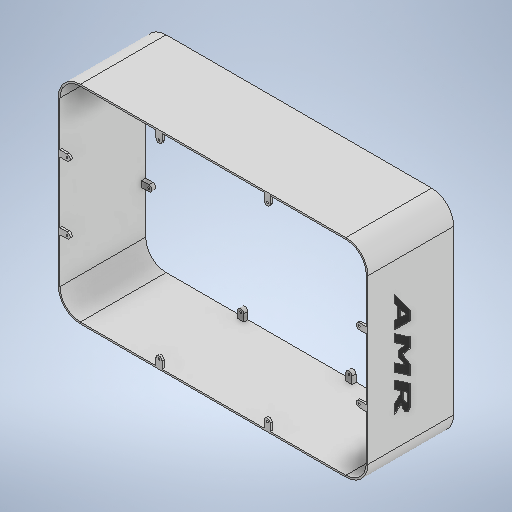
# Autodesk Inventor part: product
Saved by Autodesk Inventor 2025 (Build 290162000, 162)
## iProperties
Created: 2025-10-14
Part Number: product
Material: Generic
Document SubType Name: Modeling
Designer: hp
Density: 1 g/cm^3
Appearance: Default
Author: hp
Autodesk Inventor part; units mm, degrees
ref_plane "YZ Plane" through (0, 0, 0) normal (1, 0, 0) x (0, 1, 0)
ref_plane "XZ Plane" through (0, 0, 0) normal (0, 1, 0) x (-1, 0, 0)
ref_plane "XY Plane" through (0, 0, 0) normal (0, 0, 1) x (1, 0, 0)
sketch "Sketch1" plane through (0, 0, 0) normal (0, 0, 1) x (1, 0, 0)
  line L0 (-325, 250) -> (325, 250)
  line L1 (375, 200) -> (375, -200)
  line L2 (325, -250) -> (-325, -250)
  line L3 (-375, -200) -> (-375, 200)
  line L4 (-375, 250) -> (375, -250) construction
  line L5 (375, 250) -> (-375, -250) construction
  arc A0 (-325, 250) -> (-375, 200) centre (-325, 200) ccw
  arc A1 (-375, -200) -> (-325, -250) centre (-325, -200) ccw
  arc A2 (375, 200) -> (325, 250) centre (325, 200) ccw
  arc A3 (325, -250) -> (375, -200) centre (325, -200) ccw
  line L6 (325, 254) -> (-325, 254)
  arc A4 (-325, 254) -> (-379, 200) centre (-325, 200) ccw
  line L7 (-379, 200) -> (-379, -200)
  arc A5 (-379, -200) -> (-325, -254) centre (-325, -200) ccw
  line L8 (-325, -254) -> (325, -254)
  arc A6 (325, -254) -> (379, -200) centre (325, -200) ccw
  line L9 (379, -200) -> (379, 200)
  arc A7 (379, 200) -> (325, 254) centre (325, 200) ccw
  line L10 (-379, 200) -> (-375, 200)
  line L11 (-375, -200) -> (-379, -200)
  line L12 (379, 200) -> (375, 200)
  line L13 (379, -200) -> (375, -200)
  point P0 (0, 0)
  dimension "d66" = 5
  dimension "d0" = 750
  dimension "d2" = 50
  dimension "d3" = 50
  dimension "d4" = 4
  dimension "d75" = 500
  constraints: 28 end point, 16 point on circle, 9 point on line, 8 centre point, 8 tangent, 6 parallel, 3 perpendicular, 2 equal radius, 2 midpoint, 1 horizontal, 7 other
  measures "d0" distance of L4.end L5.end
  measures "d2" radius of A0
  measures "d3" radius of A3
  measures "d4" distance between parallel lines of L0 L6
  measures "d75" distance between parallel lines of L0 L2
extrude "Extrusion1" add sketch "Sketch1" along normal blind 210 contours A0 L10 A4 L6 A7 L12 A2 L0 | L3 L11 L7 L10 | L12 L9 L13 L1 | A1 L2 A3 L13 A6 L8 A5 L11
sketch "Sketch2" plane through (0, 0, 210) normal (0, 0, 1) x (1, 0, 0)
  line L0 (-325, 250) -> (325, 250) projected
  line L1 (-140, 250) -> (-125, 250)
  line L2 (-125, -250) -> (-140, -250)
  line L3 (125, 250) -> (140, 250)
  line L4 (140, -250) -> (125, -250)
  line L5 (-375, -200) -> (-375, 200) projected
  line L6 (375, 90) -> (375, 75)
  line L7 (-375, 75) -> (-375, 90)
  line L8 (375, 200) -> (375, -200) projected
  line L9 (375, -75) -> (375, -90)
  line L10 (325, -250) -> (-325, -250) projected
  line L11 (125, 232.5) -> (125, 250)
  line L12 (140, 250) -> (140, 232.5)
  line L13 (-125, 250) -> (-125, 232.5)
  line L14 (-140, 232.5) -> (-140, 250)
  line L15 (-375, 90) -> (-357.5, 90)
  line L16 (-357.5, 75) -> (-375, 75)
  line L17 (-375, -75) -> (-357.5, -75)
  line L18 (-357.5, -90) -> (-375, -90)
  line L19 (-140, -250) -> (-140, -232.5)
  line L20 (-125, -232.5) -> (-125, -250)
  line L21 (140, -232.5) -> (140, -250)
  line L22 (125, -250) -> (125, -232.5)
  line L23 (357.5, -75) -> (375, -75)
  line L24 (375, -90) -> (357.5, -90)
  line L25 (357.5, 90) -> (375, 90)
  line L26 (375, 75) -> (357.5, 75)
  arc A0 (-140, 232.5) -> (-125, 232.5) centre (-132.5, 232.5) ccw
  arc A1 (125, 232.5) -> (140, 232.5) centre (132.5, 232.5) ccw
  arc A2 (-357.5, 75) -> (-357.5, 90) centre (-357.5, 82.5) ccw
  arc A3 (-357.5, -90) -> (-357.5, -75) centre (-357.5, -82.5) ccw
  arc A4 (-125, -232.5) -> (-140, -232.5) centre (-132.5, -232.5) ccw
  arc A5 (140, -232.5) -> (125, -232.5) centre (132.5, -232.5) ccw
  arc A6 (357.5, -75) -> (357.5, -90) centre (357.5, -82.5) ccw
  arc A7 (357.5, 90) -> (357.5, 75) centre (357.5, 82.5) ccw
  circle A8 centre (132.5, 232.5) radius 2.5
  circle A9 centre (-132.5, 232.5) radius 2.5
  circle A10 centre (-357.5, 82.5) radius 2.5
  circle A11 centre (-357.5, -82.5) radius 2.5
  circle A12 centre (-132.5, -232.5) radius 2.5
  circle A13 centre (132.5, -232.5) radius 2.5
  circle A14 centre (357.5, -82.5) radius 2.5
  circle A15 centre (357.5, 82.5) radius 2.5
  point P0 (-132.5, -250)
  point P1 (132.5, -250)
  point P2 (-362.5, 75)
  point P3 (362.5, -75)
  point P4 (362.5, 75)
  point P5 (362.5, -90)
  point P6 (125, -187.5)
  point P7 (-140, -187.5)
  point P8 (375, -75)
  point P9 (-375, -90)
  point P10 (140, 250)
  point P11 (-125, 250)
  point P12 (-375, 82.5)
  point P13 (-132.5, -225)
  point P14 (375, -82.5)
  dimension "d32" = 750
  dimension "d33" = 15
  dimension "d48" = 0
  dimension "d50" = 250
  dimension "d51" = 235
  dimension "d53" = 15
  dimension "d54" = 15
  dimension "d55" = 150
  dimension "d56" = 160
  dimension "d57" = 15
  dimension "d58" = 150
  dimension "d59" = 160
  dimension "d60" = 15
  dimension "d61" = 15
  dimension "d62" = 250
  dimension "d63" = 250
  dimension "d64" = 15
  dimension "d65" = 5
  dimension "d66" = 5
  dimension "d67" = 5
  dimension "d68" = 5
  dimension "d69" = 5
  dimension "d70" = 5
  dimension "d71" = 5
  dimension "d72" = 5
  dimension "d76" = 17.5
  dimension "d78" = 17.5
  dimension "d79" = 17.5
  dimension "d80" = 15
  dimension "d81" = 17.5
  dimension "d82" = 17.5
  dimension "d83" = 25
  dimension "d84" = 17.5
  dimension "d85" = 17.5
  constraints: 46 end point, 19 parallel, 17 point on circle, 16 centre point, 16 tangent, 12 point on line, 8 coincident, 8 perpendicular, 6 horizontal, 4 midpoint, 1 collinear
  measures "d32" distance of L7.end L6.start
  measures "d33" distance of L6.start L6.end
  measures "d48" distance from line of L10 point (-132.5, -250)
  measures "d50" distance from line of L3.start L13
  measures "d51" distance between parallel lines of L8 L12
  measures "d53" distance from line of L3.end L11
  measures "d54" distance between parallel lines of L16 L15
  measures "d55" distance from line of L17 point (-362.5, 75)
  measures "d56" distance between parallel lines of L10 L18
  measures "d57" distance between parallel lines of L18 L17
  measures "d58" distance of point (362.5, -75) point (362.5, 75)
  measures "d59" distance from line of L10 point (362.5, -90)
  measures "d60" distance between parallel lines of L24 L23
  measures "d61" distance from line of point (125, -187.5) L21
  measures "d62" distance from line of L8 point (125, -187.5)
  measures "d63" distance between parallel lines of L22 L20
  measures "d64" distance from line of L20 point (-140, -187.5)
  measures "d65" diameter of A8
  measures "d66" diameter of A9
  measures "d67" diameter of A10
  measures "d68" diameter of A11
  measures "d69" diameter of A12
  measures "d70" diameter of A13
  measures "d71" diameter of A14
  measures "d72" diameter of A15
  measures "d76" distance from line of L4 A5.centre
  measures "d78" distance from line of A1.centre L3
  measures "d79" distance from line of A0.centre L0
  measures "d80" distance between parallel lines of L13 L14
  measures "d81" distance of point (-375, 82.5) A2.centre
  measures "d82" distance from line of L5 A3.centre
  measures "d83" distance from line of L10 point (-132.5, -225)
  measures "d84" distance of point (375, -82.5) A6.centre
  measures "d85" distance from line of A7.centre L6
extrude "Extrusion2" add sketch "Sketch2" against normal blind 5
sketch "Sketch3" plane through (379, -200, 0) normal (1, 0, 0) x (0, 0, -1)
  line L0 (-250, 400) -> (-250, -1.3337)
  line L1 (-250, -1.3337) -> (0, -1.3337)
  line L2 (0, -1.3337) -> (0, 400)
  line L3 (0, 400) -> (-250, 400)
  line L4 (0, 0) -> (0, 400) projected
  line L5 (-145, 328.6362) -> (-105, 274.3737)
  line L6 (-105, 274.3737) -> (-105, 252.4612)
  line L7 (-105, 252.4612) -> (-145, 252.6233)
  line L8 (-145, 252.6233) -> (-145, 273.304)
  line L9 (-145, 273.304) -> (-136.8314, 272.7529)
  line L10 (-136.8314, 272.7529) -> (-136.8314, 297.9393)
  line L11 (-136.8314, 297.9393) -> (-145, 308.4742)
  line L12 (-145, 308.4742) -> (-145, 328.6362)
  line L13 (-129.5705, 272.2343) -> (-116.3776, 271.4239)
  line L14 (-116.3776, 271.4239) -> (-129.5705, 288.5714)
  line L15 (-129.5705, 288.5714) -> (-129.5705, 272.2343)
  line L16 (-145, 162.8664) -> (-145, 182.8664)
  line L17 (-145, 182.8664) -> (-118.4846, 164.8437)
  line L18 (-118.4846, 164.8437) -> (-135.5997, 191.0674)
  line L19 (-135.5997, 191.0674) -> (-135.5997, 204.7789)
  line L20 (-135.5997, 204.7789) -> (-118.4846, 207.7286)
  line L21 (-118.4846, 207.7286) -> (-145, 225.7513)
  line L22 (-145, 225.7513) -> (-145, 244.6816)
  line L23 (-145, 244.6816) -> (-105, 217.4855)
  line L24 (-105, 217.4855) -> (-105, 194.2764)
  line L25 (-105, 194.2764) -> (-124.7407, 189.9653)
  line L26 (-124.7407, 189.9653) -> (-105, 158.8469)
  line L27 (-105, 158.8469) -> (-105, 135.6703)
  line L28 (-105, 135.6703) -> (-145, 162.8664)
  line L29 (-145, 72.2991) -> (-145, 96.8048)
  line L30 (-145, 96.8048) -> (-130.316, 109.1549)
  line L31 (-130.316, 109.1549) -> (-130.316, 116.351)
  line L32 (-130.316, 116.351) -> (-145, 126.3348)
  line L33 (-145, 126.3348) -> (-145, 146.3348)
  line L34 (-145, 146.3348) -> (-105, 119.1387)
  line L35 (-105, 119.1387) -> (-105, 86.9183)
  spline S0 degree 2 poles (-105, 86.9183) (-105, 80.2732) (-105.8428, 70.9377) (-107.1394, 67.6314) knots 0 0 0 1 2 2 2
  spline S1 degree 2 poles (-107.1394, 67.6314) (-108.5008, 64.2602) (-112.7472, 62.0884) (-115.9887, 64.2926) knots 0 0 0 1 2 2 2
  spline S2 degree 2 poles (-115.9887, 64.2926) (-120.5592, 67.4045) (-126.2966, 79.5925) (-127.9822, 87.6638) knots 0 0 0 1 2 2 2
  line L36 (-127.9822, 87.6638) -> (-145, 72.2991)
  spline S3 degree 2 poles (-117.2528, 85.7837) (-115.7293, 84.7789) (-113.5575, 85.6217) (-112.9741, 87.8907) knots 0 0 0 1 2 2 2
  spline S4 degree 2 poles (-112.9741, 87.8907) (-112.5851, 89.5114) (-112.3582, 93.9847) (-112.3582, 97.4207) knots 0 0 0 1 2 2 2
  line L37 (-112.3582, 97.4207) -> (-112.3582, 104.1306)
  line L38 (-112.3582, 104.1306) -> (-123.1199, 111.4563)
  line L39 (-123.1199, 111.4563) -> (-123.1199, 105.6865)
  spline S5 degree 2 poles (-123.1199, 105.6865) (-123.1199, 101.505) (-122.6013, 95.3137) (-121.7909, 92.6881) knots 0 0 0 1 2 2 2
  spline S6 degree 2 poles (-121.7909, 92.6881) (-121.013, 90.257) (-118.9384, 86.9507) (-117.2528, 85.7837) knots 0 0 0 1 2 2 2
  point P0 (0, 200)
  constraints: 1 coincident, 1 collinear, 2 other
sketch "Sketch4" plane through (0, 0, 0) normal (0, 0, -1) x (-1, 0, 0)
  line L0 (-325, 250) -> (325, 250)
  line L1 (-140, 250) -> (-125, 250)
  line L2 (-125, -250) -> (-140, -250)
  line L3 (125, 250) -> (140, 250)
  line L4 (140, -250) -> (125, -250)
  line L5 (-375, -209.7168) -> (-375, 129.8759)
  line L6 (375, 90) -> (375, 75)
  line L7 (-375, 75) -> (-375, 90)
  line L8 (375, 166.9694) -> (375, -233.0306)
  line L9 (375, -75) -> (375, -90)
  line L10 (254.1053, -250) -> (-395.8947, -250)
  line L11 (125, 232.5) -> (125, 250)
  line L12 (140, 250) -> (140, 232.5)
  line L13 (-125, 250) -> (-125, 232.5)
  line L14 (-140, 232.5) -> (-140, 250)
  line L15 (-375, 90) -> (-357.5, 90)
  line L16 (-357.5, 75) -> (-375, 75)
  line L17 (-375, -75) -> (-357.5, -75)
  line L18 (-357.5, -90) -> (-445.8947, -90)
  line L19 (-140, -250) -> (-140, -232.5)
  line L20 (-125, -232.5) -> (-125, -250)
  line L21 (140, -232.5) -> (140, -250)
  line L22 (125, -250) -> (125, -232.5)
  line L23 (357.5, -75) -> (375, -75)
  line L24 (375, -90) -> (357.5, -90)
  line L25 (357.5, 90) -> (375, 90)
  line L26 (375, 75) -> (357.5, 75)
  arc A0 (-140, 232.5) -> (-125, 232.5) centre (-132.5, 232.5) ccw
  arc A1 (125, 232.5) -> (140, 232.5) centre (132.5, 232.5) ccw
  arc A2 (-357.5, 75) -> (-357.5, 90) centre (-357.5, 82.5) ccw
  arc A3 (-357.5, -90) -> (-357.5, -75) centre (-357.5, -82.5) ccw
  arc A4 (-125, -232.5) -> (-140, -232.5) centre (-132.5, -232.5) ccw
  arc A5 (140, -232.5) -> (125, -232.5) centre (132.5, -232.5) ccw
  arc A6 (357.5, -75) -> (357.5, -90) centre (357.5, -82.5) ccw
  arc A7 (357.5, 90) -> (357.5, 75) centre (357.5, 82.5) ccw
  circle A8 centre (132.5, 232.5) radius 2.5
  circle A9 centre (-132.5, 232.5) radius 2.5
  circle A10 centre (-357.5, 82.5) radius 2.5
  circle A11 centre (-357.5, -82.5) radius 2.5
  circle A12 centre (-132.5, -232.5) radius 2.5
  circle A13 centre (132.5, -232.5) radius 2.5
  circle A14 centre (357.5, -82.5) radius 2.5
  circle A15 centre (357.5, 82.5) radius 2.5
  line L27 (375, -200) -> (375, 200) projected
  line L28 (-325, -250) -> (325, -250) projected
  line L29 (325, 250) -> (-325, 250) projected
  line L30 (-375, 200) -> (-375, -200) projected
  point P0 (0, 0)
  point P1 (-132.5, -250)
  point P2 (132.5, -250)
  point P3 (-433.3947, 75)
  point P4 (291.6053, -75)
  point P5 (291.6053, 75)
  point P6 (291.6053, -90)
  point P7 (125, -220.5306)
  point P8 (-140, -220.5306)
  point P9 (-375, 82.5)
  point P10 (-132.5, -225)
  point P11 (375, -82.5)
  point P12 (-375, -90)
  dimension "d86" = 750
  dimension "d87" = 15
  dimension "d88" = 0
  dimension "d89" = 250
  dimension "d90" = 235
  dimension "d91" = 15
  dimension "d92" = 15
  dimension "d93" = 150
  dimension "d94" = 160
  dimension "d95" = 15
  dimension "d96" = 150
  dimension "d97" = 160
  dimension "d98" = 15
  dimension "d99" = 15
  dimension "d100" = 250
  dimension "d101" = 250
  dimension "d102" = 15
  dimension "d103" = 5
  dimension "d104" = 5
  dimension "d105" = 5
  dimension "d106" = 5
  dimension "d107" = 5
  dimension "d108" = 5
  dimension "d109" = 5
  dimension "d110" = 5
  dimension "d111" = 17.5
  dimension "d112" = 17.5
  dimension "d113" = 17.5
  dimension "d114" = 15
  dimension "d115" = 17.5
  dimension "d116" = 17.5
  dimension "d117" = 25
  dimension "d118" = 17.5
  dimension "d119" = 17.5
  dimension "d120" = 375
  constraints: 54 end point, 19 parallel, 17 point on circle, 16 centre point, 16 tangent, 12 point on line, 8 coincident, 8 perpendicular, 6 horizontal, 5 collinear, 4 midpoint
  measures "d86" distance of L7.end L6.start
  measures "d87" distance of L6.start L6.end
  measures "d88" distance from line of L10 point (-132.5, -250)
  measures "d89" distance from line of L3.start L13
  measures "d90" distance between parallel lines of L8 L12
  measures "d91" distance from line of L3.end L11
  measures "d92" distance between parallel lines of L16 L15
  measures "d93" distance from line of L17 point (-433.395, 75)
  measures "d94" distance between parallel lines of L10 L18
  measures "d95" distance between parallel lines of L18 L17
  measures "d96" distance of point (291.605, -75) point (291.605, 75)
  measures "d97" distance from line of L10 point (291.605, -90)
  measures "d98" distance between parallel lines of L24 L23
  measures "d99" distance from line of point (125, -220.531) L21
  measures "d100" distance from line of L8 point (125, -220.531)
  measures "d101" distance between parallel lines of L22 L20
  measures "d102" distance from line of L20 point (-140, -220.531)
  measures "d103" diameter of A8
  measures "d104" diameter of A9
  measures "d105" diameter of A10
  measures "d106" diameter of A11
  measures "d107" diameter of A12
  measures "d108" diameter of A13
  measures "d109" diameter of A14
  measures "d110" diameter of A15
  measures "d111" distance from line of L4 A5.centre
  measures "d112" distance from line of A1.centre L3
  measures "d113" distance from line of A0.centre L0
  measures "d114" distance between parallel lines of L13 L14
  measures "d115" distance of point (-375, 82.5) A2.centre
  measures "d116" distance from line of L5 A3.centre
  measures "d117" distance from line of L10 point (-132.5, -225)
  measures "d118" distance of point (375, -82.5) A6.centre
  measures "d119" distance from line of A7.centre L6
  measures "d120" distance from line of point (0, 0) L8
extrude "Extrusion3" add sketch "Sketch4" against normal blind 10
emboss "Emboss1" sketch "Sketch3" operation cut depth 2 direction (-1, 0, 0) contours L5 L6 L7 L8 L9 L10 L11 L12 | L16 L17 L18 L19 L20 L21 L22 L23 L24 L25 L26 L27 L28 | L29 L30 L31 L32 L33 L34 L35 S0 S1 S2 L36
body "Solid1"
